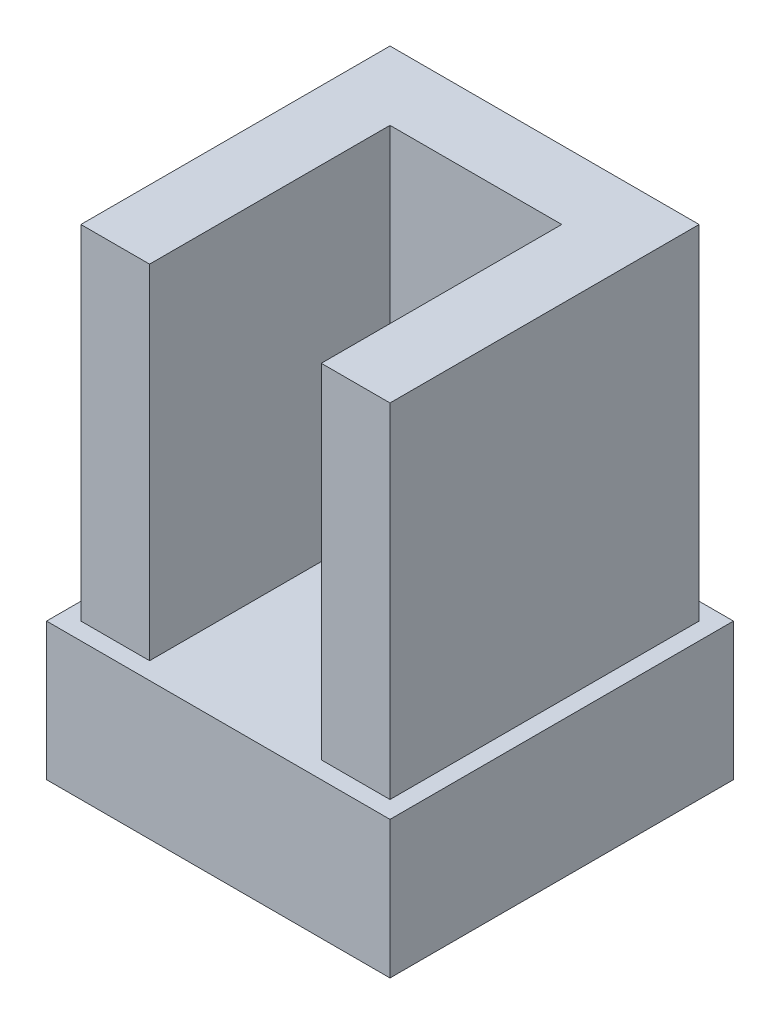
# Autodesk Inventor part: XPulleySupport
Saved by Autodesk Inventor 2019 (Build 230136000, 136)
## iProperties
Created: 2019-08-19
Part Number: XPulleySupport
Material: Generic
Document SubType Name: Modeling
Designer: Bruno
Density: 1 g/cm^3
Appearance: Default
Author: Bruno
Autodesk Inventor part; units mm, degrees
ref_plane "YZ Plane" through (0, 0, 0) normal (1, 0, 0) x (0, 1, 0)
ref_plane "XZ Plane" through (0, 0, 0) normal (0, 1, 0) x (-1, 0, 0)
ref_plane "XY Plane" through (0, 0, 0) normal (0, 0, 1) x (1, 0, 0)
sketch "Sketch2" plane through (0, 0, 0) normal (0, 1, 0) x (-1, 0, 0)
  line L0 (10.6557, -7.541) -> (-9.3443, -7.541)
  line L1 (-9.3443, -7.541) -> (-9.3443, 12.459)
  line L2 (-9.3443, 12.459) -> (10.6557, 12.459)
  line L3 (10.6557, 12.459) -> (10.6557, -7.541)
  point P0 (0, 0)
  dimension "d10" = 20
  dimension "d11" = 20
  constraints: 8 end point, 2 parallel, 1 horizontal, 1 perpendicular
  measures "d10" distance of L2.end L0.start
  measures "d11" distance of L0.start L0.end
extrude "Extrusion3" add sketch "Sketch2" along normal blind 8
sketch "Sketch3" plane through (0, 8, 0) normal (0, 1, 0) x (1, 0, 0)
  line L0 (9.3443, 7.541) -> (-10.6557, 7.541) projected
  line L1 (-10.6557, 7.541) -> (-10.6557, -12.459) projected
  line L2 (-10.6557, -12.459) -> (9.3443, -12.459) projected
  line L3 (9.3443, -12.459) -> (9.3443, 7.541) projected
  line L4 (-9.6557, -11.459) -> (-9.6557, 6.541)
  line L5 (-9.6557, 6.541) -> (8.3443, 6.541)
  line L6 (8.3443, 6.541) -> (8.3443, -11.459)
  line L7 (8.3443, -11.459) -> (4.3443, -11.459)
  line L8 (4.3443, -11.459) -> (4.3443, 2.541)
  line L9 (4.3443, 2.541) -> (-5.6557, 2.541)
  line L10 (-5.6557, 2.541) -> (-5.6557, -11.459)
  line L11 (-5.6557, -11.459) -> (-9.6557, -11.459)
  line L12 (-9.6557, 6.541) -> (-10.6557, 6.541) construction
  line L13 (8.3443, 6.541) -> (9.3443, 6.541) construction
  line L14 (-9.6557, 6.541) -> (-9.6557, 7.541) construction
  point P0 (0, 0)
  dimension "d14" = 10
  dimension "d15" = 4
  dimension "d16" = 4
  dimension "d17" = 1
  dimension "d18" = 14
  constraints: 22 end point, 9 perpendicular, 5 point on line, 2 collinear, 1 vertical
  measures "d14" distance of L8.end L9.end
  measures "d15" distance of L6.end L7.end
  measures "d16" distance between parallel lines of L5 L9
  measures "d17" distance of L4.end L14.end
  measures "d18" distance of L9.end L10.end
extrude "Extrusion4" add sketch "Sketch3" along normal blind 20 contours L4 L5 L6 L7 L8 L9 L10 L11
sketch "Sketch4" plane through (8.3443, 8, -6.541) normal (0, 0, -1) x (-1, 0, 0)
  circle A0 centre (9, 9.875) radius 2.125
  line L0 (9, 9.875) -> (0, 9.875) construction
  line L1 (0, 0) -> (0, 20) projected
  line L2 (9, 9.875) -> (18, 9.875) construction
  line L3 (18, 0) -> (18, 20) projected
  line L4 (0, 20) -> (18, 20) projected
  point P0 (8.3443, -8)
  dimension "d21" = 4.25
  dimension "d22" = 8
  constraints: 4 end point, 3 point on line, 1 centre point, 1 collinear, 1 horizontal
  measures "d21" diameter of A0
  measures "d22" distance edge to line of A0 L4
extrude "Extrusion5" cut sketch "Sketch4" against normal up to next
body "Solid2"
